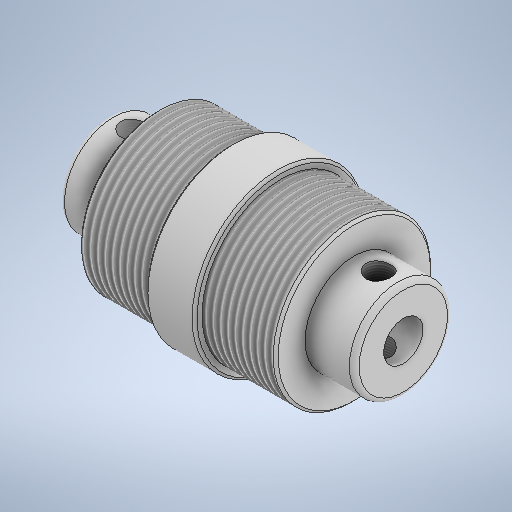
# Autodesk Inventor part: sprocet adaptor2
Saved by Autodesk Inventor 2026.1 (Build 301233020, 233B)
## iProperties
Created: 2026-01-22
Part Number: sprocet adaptor2
Material: Generic
Document SubType Name: Modeling
Designer: user
Density: 1 g/cm^3
Appearance: Default
Mass: 17.8012 g
Surface Area: 52.9443 cm^2
Volume: 17.8012 cm^3
Author: user
Autodesk Inventor part; units mm, degrees
ref_plane "XY Plane" through (0, 0, 0) normal (0, 0, 1) x (1, 0, 0)
sketch "Sketch1" plane through (0, 0, 0) normal (1, 0, 0) x (0, 1, 0)
  circle A0 centre (0, 0) radius 16
  dimension "d0" = 32
  constraints: 1 centre point, 1 coincident
  measures "d0" diameter of A0
extrude "Extrusion1" add sketch "Sketch1" along normal blind 15
sketch "Sketch2" plane through (15, 0, 0) normal (1, 0, 0) x (0, 0, -1)
  circle A0 centre (0, 0) radius 17.5
  dimension "d3" = 35
  constraints: 1 centre point, 1 coincident
  measures "d3" diameter of A0
extrude "Extrusion2" add sketch "Sketch2" along normal blind 10
ref_plane "Work Plane2" through (20, 0, 0) normal (1, 0, 0) x (0, 1, 0)
mirror "Mirror1" about plane through (20, 0, 0) normal (1, 0, 0) of "Extrusion1"
thread "Thread3" size "M32x1.5" class "6g" standard "ANSI Metric M Profile" length 20
thread "Thread4" size "M32x1.5" class "6g" standard "ANSI Metric M Profile" length 20
chamfer "Chamfer2" distance 0.5 angle 45 2 edges at (15, 0, 17.5) (25, 0, 17.5)
sketch "Sketch6" plane through (40, 0, 0) normal (1, 0, 0) x (0, 0, -1)
  circle A0 centre (0, 0) radius 10
  dimension "d33" = 20
  constraints: 1 centre point, 1 coincident
  measures "d33" diameter of A0
extrude "Extrusion6" add sketch "Sketch6" along normal blind 10
ref_plane "Work Plane3" through (0, 10, 0) normal (0, 1, 0) x (-1, 0, 0)
sketch "Sketch8" plane through (0, 10, 0) normal (0, 1, 0) x (-1, 0, 0)
  line L0 (-50, 10) -> (-50, -10) projected
  line L1 (-50, 0) -> (-45, 0)
  circle A0 centre (-45, 0) radius 2.5
  point P0 (0, 0)
  dimension "d40" = 5
  dimension "d41" = 5
  constraints: 2 end point, 1 centre point, 1 coincident, 1 horizontal, 1 midpoint
  measures "d40" distance of L1.start L1.end
  measures "d41" diameter of A0
extrude "Extrusion8" cut sketch "Sketch8" against normal blind 30
mirror "Mirror2" about plane through (20, 0, 0) normal (1, 0, 0) of "Extrusion6", "Extrusion8"
sketch "Sketch7" plane through (50, 0, 0) normal (1, 0, 0) x (0, 0, -1)
  circle A0 centre (0, 0) radius 4
  dimension "d36" = 8
  constraints: 1 centre point, 1 coincident
  measures "d36" diameter of A0
extrude "Extrusion7" cut sketch "Sketch7" against normal blind 73
chamfer "Chamfer3" distance 0.5 angle 45 2 edges at (40, -16, 0) (0, -16, 0)
fillet "Fillet3" radius 1 2 edges at (50, 0, 10) (-10, 0, 10)
thread "Thread5" size "M5x0.5" class "6H" standard "ANSI Metric M Profile" length 20
thread "Thread6" size "M5x0.5" class "6H" standard "ANSI Metric M Profile" length 20
body "Solid1"
